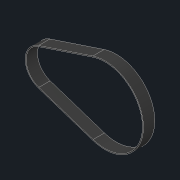
# Autodesk Inventor part: belt5
Saved by Autodesk Inventor 2022 (Build 260153000, 153)
## iProperties
Created: 2021-08-06
Part Number: belt5
Material: ゴム
Document SubType Name: Modeling
Designer: yuta0
Density: 0.93 g/cm^3
Appearance: ゴム - 黒
購入先: ミスミ
在庫数: 0.0
Author: yuta0
Autodesk Inventor part; units mm, degrees
ref_plane "YZ Plane" through (0, 0, 0) normal (1, 0, 0) x (0, 1, 0)
ref_plane "XZ Plane" through (0, 0, 0) normal (0, 1, 0) x (-1, 0, 0)
ref_plane "XY Plane" through (0, 0, 0) normal (0, 0, 1) x (1, 0, 0)
sketch "スケッチ1" plane through (0, 0, 0) normal (0, 0, 1) x (1, 0, 0)
  arc A0 (-5.2692, 15.8588) -> (-5.2692, -15.8588) centre (0, 0) ccw
  arc A1 (42.4616, -31.7176) -> (42.4616, 31.7176) centre (53, 0) ccw
  line L0 (-5.2692, 15.8588) -> (42.4616, 31.7176)
  line L1 (-5.2692, -15.8588) -> (42.4616, -31.7176)
  line L2 (42.3295, 32.1153) -> (-5.4013, 16.2564)
  arc A2 (-5.4013, 16.2564) -> (-5.4013, -16.2564) centre (0, 0) ccw
  line L3 (-5.4013, -16.2564) -> (42.3295, -32.1153)
  arc A3 (42.3295, -32.1153) -> (42.3295, 32.1153) centre (53, 0) ccw
  line L4 (42.5818, 31.3561) -> (-5.149, 15.4973)
  arc A4 (-5.149, 15.4973) -> (-5.149, -15.4973) centre (0, 0) ccw
  line L5 (-5.149, -15.4973) -> (42.5818, -31.3561)
  arc A5 (42.5818, -31.3561) -> (42.5818, 31.3561) centre (53, 0) ccw
  dimension "d6" = 33.4225
  dimension "d7" = 66.8451
  dimension "d8" = 53
  dimension "d11" = 0.419
  dimension "d12" = 0.8
  constraints: 12 end point, 12 point on circle, 6 centre point, 4 tangent, 1 coincident, 1 horizontal alignment, 6 other
  measures "d6" diameter of A0
  measures "d7" diameter of A1
  measures "d8" distance of A1.centre A0.centre
  measures "d11" distance between parallel lines of L0 L2
  measures "d12" distance between parallel lines of L2 L4
extrude "押し出し1" add sketch "スケッチ1" along normal mid plane 10 contours L0 A1 L1 A0 | A3 L3 A2 L2
